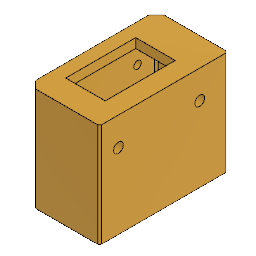
switch_mount v5 (Autodesk Fusion 360 design; units mm, degrees)
Autodesk Fusion 360 part; units mm, degrees
sketch "Sketch1" plane through (0, 0, 0) normal (0, 0, 1) x (1, 0, 0)
  line L0 (10.5, -18.575) -> (-10.5, -18.575)
  line L1 (-10.5, -18.575) -> (-10.5, 18.575)
  line L2 (-10.5, 18.575) -> (10.5, 18.575)
  line L3 (10.5, 18.575) -> (10.5, -18.575)
  line L4 (10.5, -18.575) -> (-10.5, 18.575) construction
  line L5 (-10.5, -18.575) -> (10.5, 18.575) construction
  line L6 (15.5, -26.575) -> (-12.5, -26.575)
  line L7 (-12.5, -26.575) -> (-12.5, 31.575)
  line L8 (-12.5, 31.575) -> (15.5, 31.575)
  line L9 (15.5, 31.575) -> (15.5, -26.575)
  line L10 (20.5, -31.575) -> (-17.5, -31.575)
  line L11 (-17.5, -31.575) -> (-17.5, 36.575)
  line L12 (-17.5, 36.575) -> (20.5, 36.575)
  line L13 (20.5, 36.575) -> (20.5, -31.575)
  dimension "d1" = 21
  dimension "d2" = 37.15
  dimension "d4" = 2
  dimension "d5" = 8
  dimension "d6" = 5
  dimension "d7" = 5
  dimension "d19" = 13
  dimension "d20" = 5
  dimension "d21" = 5
  dimension "d22" = 5
  constraint perpendicular L0 L1
  constraint parallel L0 L2
  constraint parallel L1 L3
  constraint horizontal L0
  constraint coincident L4 origin
  constraint coincident L5 origin
  constraint perpendicular L6 L7
  constraint parallel L6 L8
  constraint parallel L7 L9
  constraint horizontal L6
  constraint perpendicular L10 L11
  constraint parallel L10 L12
  constraint parallel L11 L13
  constraint horizontal L10
  measures "d1" distance of L1.end L2.end
  measures "d2" distance of L0 L2
  measures "d4" distance of L1 L7
  measures "d5" distance of L0 L6
  measures "d6" distance of L7 L11
  measures "d7" distance of L6 L10
  measures "d19" distance of L2 L8
  measures "d20" distance of L3 L9
  measures "d21" distance of L8 L12
  measures "d22" distance of L9 L13
  measures "d30" diameter of L0.end
extrude "Extrude1" add sketch "Sketch1" against normal blind 5 contours L6 L7 L8 L9
extrude "Extrude2" add sketch "Sketch1" against normal blind 55 contours L10 L11 L12 L13
sketch "Sketch3" plane through (20.5, 0, 0) normal (1, 0, 0) x (0, 1, 0)
  line L0 (36.575, 0) -> (-31.575, 0)
  line L1 (-31.575, 0) -> (-31.575, -55)
  line L2 (-31.575, -55) -> (36.575, -55)
  line L3 (36.575, -55) -> (36.575, 0)
  line L4 (-31.575, -15) -> (36.575, -15) construction
  line L5 (36.575, 0) -> (-31.575, 0)
  circle A0 centre (21.575, -15) radius 2.6
  circle A1 centre (-21.575, -15) radius 2.6
  line L6 (-26.575, -5) -> (31.575, -5)
  line L7 (31.575, -5) -> (31.575, -55)
  line L8 (31.575, -55) -> (-26.575, -55)
  line L9 (-26.575, -55) -> (-26.575, -5)
  dimension "d23" = 15
  dimension "d24" = 5.2
  dimension "d25" = 5.2
  dimension "d26" = 10
  dimension "d27" = 5
  constraint coincident L1 L4.start
  constraint coincident L3 L4.end
  constraint perpendicular L3 L4
  constraint coincident L4 A0.centre
  constraint coincident L4 A1.centre
  measures "d23" distance of L4 L5
  measures "d24" diameter of A0
  measures "d25" diameter of A1
  measures "d26" distance of A0.centre L7
  measures "d27" distance of A1.centre L9
extrude "Extrude4" cut sketch "Sketch3" against normal up to surface (5 mm away) contours A0 | A1
sketch "Sketch4" plane through (-17.5, 0, 0) normal (-1, 0, 0) x (0, -1, 0)
  line L0 (31.575, 0) -> (-36.575, 0)
  line L1 (-36.575, 0) -> (-36.575, -55)
  line L2 (-36.575, -55) -> (31.575, -55)
  line L3 (31.575, -55) -> (31.575, 0)
  circle A0 centre (21.575, -15) radius 2.6
  circle A1 centre (-21.575, -15) radius 2.6
  line L4 (26.575, -5) -> (-31.575, -5)
  line L5 (-31.575, -5) -> (-31.575, -55)
  line L6 (-31.575, -55) -> (26.575, -55)
  line L7 (26.575, -55) -> (26.575, -5)
  circle A2 centre (-21.575, -15) radius 2
  circle A3 centre (21.575, -15) radius 2
  dimension "d30" = 4
  dimension "d31" = 4
  constraint concentric A1 A2
  constraint concentric A0 A3
  measures "d30" diameter of A2
  measures "d31" diameter of A3
chamfer "Chamfer5" distance 1 angle 45 2 edges at (-12.5, -26.575, -30) (-12.5, 31.575, -30)
extrude "Extrude5" cut sketch "Sketch4" against normal through all contours A2 | A3
sketch "Sketch5" plane through (0, 36.575, 0) normal (0, 1, 0) x (-1, 0, 0)
  line L0 (-20.5, -55) -> (17.5, -55)
  line L1 (17.5, 0) -> (-20.5, 0)
  line L2 (-1.5, -55) -> (-1.5, 0) construction
  line L3 (2, -47) -> (4, -47)
  line L4 (4, -47) -> (4, -53)
  line L5 (4, -53) -> (2, -53)
  line L6 (2, -53) -> (2, -47)
  line L7 (-7, -47) -> (-7, -53)
  line L8 (-7, -53) -> (-5, -53)
  line L9 (-5, -53) -> (-5, -47)
  line L10 (-5, -47) -> (-7, -47)
  line L11 (17.5, -55) -> (17.5, 0)
  line L12 (-20.5, 0) -> (-20.5, -55)
  dimension "d35" = 6
  dimension "d36" = 2
  dimension "d37" = 3.5
  dimension "d38" = 2
  constraint midpoint L0 L2.start
  constraint midpoint L1 L2.end
  constraint horizontal L3
  constraint vertical L4
  constraint horizontal L5
  constraint vertical L6
  constraint symmetric L2 L3.start L9.end
  constraint symmetric L2 L3.end L7.start
  constraint symmetric L2 L4.end L7.end
  constraint symmetric L2 L5.end L8.end
  measures "d35" distance of L3.end L4.end
  measures "d36" distance of L3.start L3.end
  measures "d37" distance of L2 L6
  measures "d38" distance of L0 L5
extrude "Extrude6" cut sketch "Sketch5" against normal up to surface (5 mm away) contours L3 L4 L5 L6 | L7 L8 L9 L10
chamfer "Chamfer2" distance 1 angle 45 2 edges at (5, 31.575, -50) (-2, 31.575, -50)
chamfer "Chamfer3" distance 1 angle 45 2 edges at (5, 36.575, -50) (-2, 36.575, -50)
chamfer "Chamfer4" distance 1 angle 45 1 edges at (1.5, 31.575, -55)
chamfer "Chamfer1" distance 1 angle 45 2 edges at (20.5, 36.575, -27.5) (20.5, -31.575, -27.5)
chamfer "Chamfer6" distance 4 angle 45 2 edges at (-17.5, 36.575, -27.5) (-17.5, -31.575, -27.5)
equation "d30 = d31"
